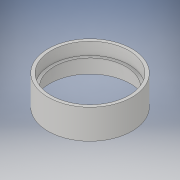
# Autodesk Inventor part: Aluminum Skirt 8-inch v1
Saved by Autodesk Inventor 2017 (Build 210142000, 142)
## iProperties
Created: 2016-07-08
Part Number: Aluminum Skirt 8-inch v1
Material: Generic
Document SubType Name: Modeling
Designer: Bill
Density: 1 g/cm^3
Appearance: Default
Author: Bill
Autodesk Inventor part; units mm, degrees
ref_plane "YZ Plane" through (0, 0, 0) normal (1, 0, 0) x (0, 1, 0)
ref_plane "XZ Plane" through (0, 0, 0) normal (0, 1, 0) x (-1, 0, 0)
ref_plane "XY Plane" through (0, 0, 0) normal (0, 0, 1) x (1, 0, 0)
sketch "Sketch1" plane through (0, 0, 0) normal (0, 0, 1) x (1, 0, 0)
  line L0 (-86.7918, 10.7122) -> (-80.4418, 10.7122)
  line L1 (-80.4418, 10.7122) -> (-80.4418, -14.7)
  line L2 (-80.4418, -14.7) -> (-74.0918, -14.7)
  line L3 (-86.7918, -50.2478) -> (-86.7918, 10.7122)
  line L4 (-86.7918, -50.2478) -> (-83.6168, -50.2478)
  line L5 (-83.6168, -50.2478) -> (-74.0918, -14.7)
  line L6 (0, -62.4398) -> (0, 22.9042) projected
  point P0 (0, 0)
  dimension "d0" = 6.35
  dimension "d1" = 6.35
  dimension "d2" = 3.175
  dimension "d3" = 105
  dimension "d4" = 60.96
  dimension "d5" = 86.7918
  constraints: 12 end point, 2 horizontal, 2 perpendicular, 1 parallel
  measures "d0" distance of L0.start L0.end
  measures "d1" distance of L1.end L2.end
  measures "d2" distance of L3.start L4.end
  measures "d3" angle of L4 L5
  measures "d4" distance of L3.start L0.start
  measures "d5" distance from line of point (0, 0) L3
revolve "Revolution1" add sketch "Sketch1" angle 360 about axis through (0, -10, 0) along (0, 1, 0)
body "Solid1"
